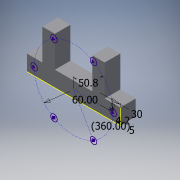
# Autodesk Inventor part: Stopper Screw Point
Saved by Autodesk Inventor 2019.4 (Build 234330000, 330)
## iProperties
Created: 2020-03-12
Part Number: Stopper Screw Point
Material: Generic
Document SubType Name: Modeling
Designer: Mark
Density: 1 g/cm^3
Appearance: Default
Author: Mark
Autodesk Inventor part; units mm, degrees
ref_plane "YZ Plane" through (0, 0, 0) normal (1, 0, 0) x (0, 1, 0)
ref_plane "XZ Plane" through (0, 0, 0) normal (0, 1, 0) x (-1, 0, 0)
ref_plane "XY Plane" through (0, 0, 0) normal (0, 0, 1) x (1, 0, 0)
sketch "Sketch1" plane through (0, 0, 0) normal (0, 0, 1) x (1, 0, 0)
  line L0 (0, 0) -> (60, 0)
  line L1 (60, 0) -> (60, 10)
  line L2 (60, 10) -> (0, 10)
  line L3 (0, 10) -> (0, 0)
  line L4 (13.3, 10) -> (21.3, 10)
  line L5 (21.3, 10) -> (21.3, 32)
  line L6 (21.3, 32) -> (13.3, 32)
  line L7 (13.3, 32) -> (13.3, 10)
  line L8 (46.7, 10) -> (38.7, 10)
  line L9 (38.7, 10) -> (38.7, 32)
  line L10 (38.7, 32) -> (46.7, 32)
  line L11 (46.7, 32) -> (46.7, 10)
  dimension "d0" = 60
  dimension "d1" = 10
  dimension "d13" = 8
  dimension "d14" = 22
  dimension "d15" = 8
  dimension "d16" = 22
  dimension "d17" = 13.3
  dimension "d18" = 13.3
  constraints: 24 end point, 6 parallel, 3 horizontal, 3 perpendicular, 2 point on line
  measures "d0" distance of L2.end L1.end
  measures "d1" distance of L1.end L0.end
  measures "d13" distance of L6.end L5.end
  measures "d14" distance of L5.end L4.end
  measures "d15" distance of L9.end L10.end
  measures "d16" distance of L8.end L9.end
  measures "d17" distance between parallel lines of L3 L7
  measures "d18" distance between parallel lines of L1 L11
extrude "Extrusion1" add sketch "Sketch1" along normal blind 10
sketch "Sketch2" plane through (0, 0, 10) normal (0, 0, 1) x (1, 0, 0)
  circle A0 centre (30, 5) radius 25.4 construction
  line L0 (60, 0) -> (60, 10) projected
  line L1 (0, 0) -> (60, 0) projected
  circle A1 centre (55.4, 5) radius 2.1
  circle A2 centre (42.7, 26.997) radius 2.1
  circle A3 centre (17.3, 26.997) radius 2.1
  circle A4 centre (4.6, 5) radius 2.1
  circle A5 centre (17.3, -16.997) radius 2.1
  circle A6 centre (42.7, -16.997) radius 2.1
  line L2 (30, 5) -> (42.7, -16.997) construction
  line L3 (30, 5) -> (55.4, 5) construction
  dimension "d4" = 50.8
  dimension "d5" = 30
  dimension "d6" = 5
  dimension "d7" = 4.2
  dimension "d10" = 360
  dimension "d12" = 60
  constraints: 7 centre point, 4 end point, 2 point on circle, 1 equal length, 1 horizontal, 1 point on line, 13 other
  measures "d4" diameter of A0
  measures "d5" distance from line of L0 L2.start
  measures "d6" distance from line of L1 L2.start
  measures "d7" diameter of A1
  measures "d12" angle of L2 L3
extrude "Extrusion2" cut sketch "Sketch2" against normal blind 10 contours A1 | A2 | A3 | A4
sketch "Sketch3" plane through (21.3, 10, 0) normal (0, 1, 0) x (1, 0, 0)
  circle A0 centre (8.7, -5) radius 3.4
  line L0 (17.4, 0) -> (0, 0) projected
  line L1 (-21.3, 0) -> (-21.3, -10) projected
  dimension "d21" = 6.8
  dimension "d22" = 5
  dimension "d23" = 30
  constraints: 1 centre point
  measures "d21" diameter of A0
  measures "d22" distance from line of L0 A0.centre
  measures "d23" distance from line of L1 A0.centre
extrude "Extrusion3" cut sketch "Sketch3" against normal up to next
fillet "Fillet1" radius 9 2 edges at (46.7, 10, 5) (13.3, 10, 5)
body "Solid1"
